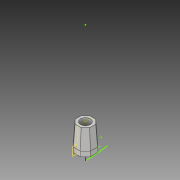
# Autodesk Inventor part: V1.0
Saved by Autodesk Inventor 2018.2 (Build 222227000, 227)
## iProperties
Created: 2018-02-16
Part Number: V1.0
Material: Generic
Document SubType Name: Modeling
Designer: Rus
Density: 1 g/cm^3
Appearance: Default
Author: Rus
Autodesk Inventor part; units mm, degrees
ref_plane "YZ Plane" through (0, 0, 0) normal (1, 0, 0) x (0, 1, 0)
ref_plane "XZ Plane" through (0, 0, 0) normal (0, 1, 0) x (-1, 0, 0)
ref_plane "XY Plane" through (0, 0, 0) normal (0, 0, 1) x (1, 0, 0)
sketch "Sketch1" plane through (0, 0, 0) normal (0, 1, 0) x (-1, 0, 0)
  line L0 (7.8908, 19.05) -> (19.05, 7.8908)
  line L1 (19.05, 7.8908) -> (19.05, -7.8908)
  line L2 (19.05, -7.8908) -> (7.8908, -19.05)
  line L3 (7.8908, -19.05) -> (-7.8908, -19.05)
  line L4 (-7.8908, -19.05) -> (-19.05, -7.8908)
  line L5 (-19.05, -7.8908) -> (-19.05, 7.8908)
  line L6 (-19.05, 7.8908) -> (-7.8908, 19.05)
  line L7 (-7.8908, 19.05) -> (7.8908, 19.05)
  point P0 (0, 0)
  point P1 (0, 0)
  dimension "d5" = 19.05
  constraints: 16 end point, 1 coincident, 1 vertical, 17 other
  measures "d5" distance from line of L1 point (0, 0)
extrude "Extrusion1" add sketch "Sketch1" against normal blind 50.8
sketch "Sketch4" plane through (0, -50.8, 0) normal (0, -1, 0) x (1, 0, 0)
  line L0 (9.2059, 22.225) -> (22.225, 9.2059)
  line L1 (22.225, 9.2059) -> (22.225, -9.2059)
  line L2 (22.225, -9.2059) -> (9.2059, -22.225)
  line L3 (9.2059, -22.225) -> (-9.2059, -22.225)
  line L4 (-9.2059, -22.225) -> (-22.225, -9.2059)
  line L5 (-22.225, -9.2059) -> (-22.225, 9.2059)
  line L6 (-22.225, 9.2059) -> (-9.2059, 22.225)
  line L7 (-9.2059, 22.225) -> (9.2059, 22.225)
  line L8 (7.8908, 19.05) -> (-7.8908, 19.05) projected
  point P0 (0, 0)
  point P1 (0, 0)
  dimension "d17" = 3.175
  constraints: 16 end point, 1 coincident, 17 other
  measures "d17" distance between parallel lines of L7 L8
loft "Loft1" add profiles "Sketch4" section 2 edges at (-13.4704, 0, 13.4704) (0, 0, 19.05) (13.4704, 0, 13.4704) (19.05, 0, 0) (13.4704, 0, -13.4704) (0, 0, -19.05) (-13.4704, 0, -13.4704) (-19.05, 0, 0)
sketch "Sketch5" plane through (0, 0, 0) normal (0, 1, 0) x (1, 0, 0)
  circle A0 centre (0, 0) radius 12.7
  dimension "d11" = 25.4
  constraints: 1 centre point, 1 coincident
  measures "d11" diameter of A0
extrude "Extrusion2" cut sketch "Sketch5" against normal blind 50.8
ref_plane "Work Plane1" through (0, -50.8, 22.225) normal (1, 0, 0) x (0, 1, 0)
sketch "Sketch6" plane through (0, -50.8, 22.225) normal (1, 0, 0) x (0, 1, 0)
  point P0 (50.8, -22.225)
sketch "Sketch7" plane through (0, -50.8, 22.225) normal (1, 0, 0) x (0, 1, 0)
  point P0 (50.8, -22.225)
sketch "Sketch8" plane through (0, -50.8, 0) normal (0, -1, 0) x (1, 0, 0)
  circle A0 centre (0, 0) radius 12.7 projected
  line L0 (9.2059, 22.225) -> (22.225, 9.2059) projected
  line L1 (-9.2059, 22.225) -> (9.2059, 22.225) projected
  line L2 (-22.225, 9.2059) -> (-9.2059, 22.225) projected
  line L3 (-22.225, -9.2059) -> (-22.225, 9.2059) projected
  line L4 (-9.2059, -22.225) -> (-22.225, -9.2059) projected
  line L5 (9.2059, -22.225) -> (-9.2059, -22.225) projected
  line L6 (22.225, -9.2059) -> (9.2059, -22.225) projected
  line L7 (22.225, 9.2059) -> (22.225, -9.2059) projected
extrude "Extrusion3" add sketch "Sketch8" along normal blind 12.7 contours A0 | L0 L7 L6 L5 L4 L3 L2 L1
sketch "Sketch9" plane through (0, -50.8, 22.225) normal (1, 0, 0) x (0, 1, 0)
  line L0 (-12.7, -31.4309) -> (-12.7, -44.45) construction
  line L1 (-12.7, -13.0191) -> (-12.7, -31.4309) construction
  line L2 (-12.7, 0) -> (-12.7, -13.0191) construction
  line L3 (0, -44.45) -> (-12.7, -44.45) construction
  line L4 (0, -44.45) -> (50.8, -41.275) construction
  line L5 (0, 0) -> (-12.7, 0) construction
  line L6 (0, 0) -> (50.8, -3.175) construction
  line L7 (0, -13.0191) -> (0, 0) construction
  line L8 (0, -34.925) -> (0, -9.525) construction
  line L9 (0, -44.45) -> (0, -31.4309) construction
  line L10 (50.8, -30.1158) -> (50.8, -41.275) construction
  line L11 (50.8, -9.525) -> (50.8, -34.925) construction
  line L12 (50.8, -3.175) -> (50.8, -14.3342) construction
  line L13 (-6.35, 0) -> (-6.35, -44.45) construction
  line L14 (-12.7, -22.225) -> (0, -22.225) construction
  arc A0 (-37.0757, -22.225) -> (-31.6983, -79.4354) centre (269.9482, -22.225) ccw
  line L15 (-37.0757, -22.225) -> (-6.35, -22.225)
  arc A1 (-6.35, -44.45) -> (-24.1759, -60.6977) centre (-5.386, -63.4102) ccw
  point P0 (50.8, -22.225)
  constraints: 6 end point, 5 midpoint, 4 point on circle, 2 centre point, 1 line through centre, 1 perpendicular
body "Solid1"
